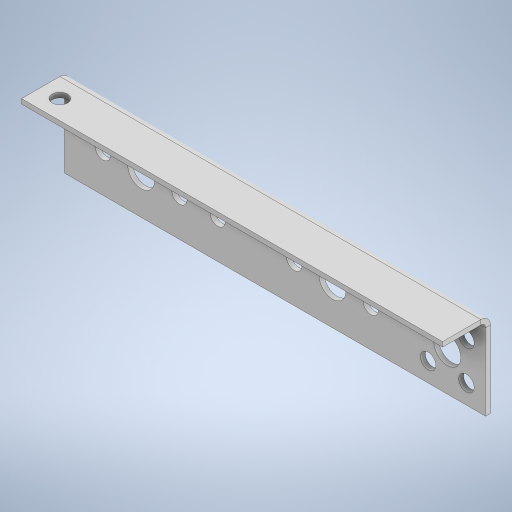
# Autodesk Inventor part: poly1
Saved by Autodesk Inventor 2023.4 (Build 274418000, 418)
## iProperties
Created: 2023-12-19
Part Number: poly1
Material: Generic
Document SubType Name: Sheet Metal
Designer: Meer
Density: 1 g/cm^3
Sheet Metal Rule: Default
Appearance: Default
Author: Meer
Autodesk Inventor part; units mm, degrees
ref_plane "YZ Plane" through (0, 0, 0) normal (1, 0, 0) x (0, 1, 0)
ref_plane "XZ Plane" through (0, 0, 0) normal (0, 1, 0) x (-1, 0, 0)
ref_plane "XY Plane" through (0, 0, 0) normal (0, 0, 1) x (1, 0, 0)
sketch "Sketch1" plane through (0, 0, 0) normal (0, 0, 1) x (1, 0, 0)
  line L0 (0, 0) -> (139.7, 0)
  line L1 (139.7, 0) -> (139.7, 25.4)
  line L2 (139.7, 25.4) -> (0, 25.4)
  line L3 (0, 25.4) -> (0, 0)
  circle A0 centre (12.7, 12.7) radius 2.54
  circle A1 centre (25.4, 12.7) radius 4.445
  circle A2 centre (38.1, 12.7) radius 2.54
  circle A3 centre (50.8, 12.7) radius 2.54
  circle A4 centre (76.2, 12.7) radius 2.54
  circle A5 centre (88.9, 12.7) radius 4.445
  circle A6 centre (101.6, 12.7) radius 2.54
  circle A7 centre (127, 12.7) radius 4.445
  circle A8 centre (133.35, 6.35) radius 2.54
  circle A9 centre (120.65, 19.05) radius 2.54
  circle A10 centre (133.35, 19.05) radius 2.54
  circle A11 centre (120.65, 6.35) radius 2.54
  dimension "d0" = 139.7
  dimension "d1" = 25.4
  dimension "d9" = 5.08
  dimension "d11" = 8.89
  dimension "d13" = 5.08
  dimension "d15" = 5.08
  dimension "d17" = 5.08
  dimension "d19" = 8.89
  dimension "d21" = 5.08
  dimension "d23" = 8.89
  dimension "d39" = 5.08
  dimension "d42" = 5.08
  dimension "d43" = 5.08
  dimension "d44" = 5.08
  measures "d0" distance of L1.end L2.end
  measures "d1" distance of L0.end L1.end
  measures "d9" diameter of A0
  measures "d11" diameter of A1
  measures "d13" diameter of A2
  measures "d15" diameter of A3
  measures "d17" diameter of A4
  measures "d19" diameter of A5
  measures "d21" diameter of A6
  measures "d23" diameter of A7
  measures "d39" diameter of A8
  measures "d42" diameter of A9
  measures "d43" diameter of A10
  measures "d44" diameter of A11
extrude "Plate4" add sketch "Sketch1" along normal blind 1.5875
sketch "Sketch6" plane through (0, 26.9875, 3.175) normal (0, 1, 0) x (-1, 0, 0)
  line L0 (-139.7, 0) -> (0, 0)
  line L1 (0, 0) -> (0, 12.7)
  line L2 (0, 12.7) -> (-139.7, 12.7)
  line L3 (-139.7, 12.7) -> (-139.7, 0)
  constraints: 6 end point, 1 horizontal, 1 perpendicular, 1 vertical
edge flange "Flange2" height 15.875 angle 90 thickness 1.5875 bend radius 1.5875 thickness toward (0, 1, 0) relief tear relief width 1.5875 relief depth 0.7937 edges at (69.85, 25.4, 1.5875) wall of the first edge with corners at (139.7, 26.9875, 3.175) (0, 26.9875, 3.175) (0, 26.9875, 15.875) (139.7, 26.9875, 15.875)
bend "Bend2"
corner "Corner2"
sketch "Sketch8" plane through (0, 28.575, 15.875) normal (0, 1, 0) x (1, 0, 0)
  line L0 (139.7, 12.7) -> (0, 12.7) projected
  line L1 (0, 12.7) -> (0, 6.35)
  line L2 (0, 0) -> (0, 12.7) projected
  line L3 (0, 6.35) -> (6.35, 6.35)
  circle A0 centre (6.35, 6.35) radius 2.54
  point P0 (0, 15.875)
  dimension "d69" = 6.35
  dimension "d70" = 5.08
  constraints: 4 end point, 1 centre point, 1 coincident, 1 midpoint, 1 perpendicular
  measures "d69" distance of L1.end L3.end
  measures "d70" diameter of A0
extrude "Extrusion1" cut sketch "Sketch8" against normal blind 1.5875
equation "\"d58\" = Thickness"
equation "\"d59\" = BendReliefWidth"
equation "\"d60\" = BendReliefDepth"
equation "\"d61\" = MinimumRemnant"
equation "\"d62\" = TransitionRadius"
equation "\"d65\" = BendRadius"
equation "\"d66\" = CornerReliefSize"
equation "\"d67\" = GapSize"
equation "\"d68\" = JacobiRadiusSize"
equation "\"BendRadius\" = Thickness"
equation "\"BendReliefWidth\" = Thickness"
equation "\"BendReliefDepth\" = 0.5 * Thickness"
equation "\"CornerReliefSize\" = 4 * Thickness"
equation "\"MinimumRemnant\" = 2 * Thickness"
equation "\"TransitionRadius\" = BendRadius"
equation "\"JacobiRadiusSize\" = BendRadius"
equation "\"GapSize\" = Thickness"
equation "\"Thickness\" = 1.5875"
body "Solid3"
